Autodesk Fusion 360 part; units mm, degrees
note: some values were not read from the file. Set by a fixed rule: which sketch regions a step uses.
(part 2 of 3)
  line L723 (-61, -7.5056) -> (-66, -4.6188)
  line L724 (-61, -13.2791) -> (-61, -7.5056)
  line L725 (-71, -7.5056) -> (-71, -13.2791)
  line L726 (-71, -13.2791) -> (-66, -16.1658)
  line L727 (-66, -16.1658) -> (-61, -13.2791)
  line L728 (-54, -4.6188) -> (-59, -7.5056)
  line L729 (-49, -7.5056) -> (-54, -4.6188)
  line L730 (-49, -13.2791) -> (-49, -7.5056)
  line L731 (-59, -7.5056) -> (-59, -13.2791)
  line L732 (-59, -13.2791) -> (-54, -16.1658)
  line L733 (-54, -16.1658) -> (-49, -13.2791)
  line L734 (-42, -4.6188) -> (-47, -7.5056)
  line L735 (-37, -7.5056) -> (-42, -4.6188)
  line L736 (-37, -13.2791) -> (-37, -7.5056)
  line L737 (-47, -7.5056) -> (-47, -13.2791)
  line L738 (-47, -13.2791) -> (-42, -16.1658)
  line L739 (-42, -16.1658) -> (-37, -13.2791)
  line L740 (-30, -4.6188) -> (-35, -7.5056)
  line L741 (-25, -7.5056) -> (-30, -4.6188)
  line L742 (-25, -13.2791) -> (-25, -7.5056)
  line L743 (-35, -7.5056) -> (-35, -13.2791)
  line L744 (-35, -13.2791) -> (-30, -16.1658)
  line L745 (-30, -16.1658) -> (-25, -13.2791)
  line L746 (-18, -4.6188) -> (-23, -7.5056)
  line L747 (-13, -7.5056) -> (-18, -4.6188)
  line L748 (-13, -13.2791) -> (-13, -7.5056)
  line L749 (-23, -7.5056) -> (-23, -13.2791)
  line L750 (-23, -13.2791) -> (-18, -16.1658)
  line L751 (-18, -16.1658) -> (-13, -13.2791)
  line L752 (-6, -4.6188) -> (-11, -7.5056)
  line L753 (-1, -7.5056) -> (-6, -4.6188)
  line L754 (-1, -13.2791) -> (-1, -7.5056)
  line L755 (-11, -7.5056) -> (-11, -13.2791)
  line L756 (-11, -13.2791) -> (-6, -16.1658)
  line L757 (-6, -16.1658) -> (-1, -13.2791)
  line L758 (6, -4.6188) -> (1, -7.5056)
  line L759 (11, -7.5056) -> (6, -4.6188)
  line L760 (11, -13.2791) -> (11, -7.5056)
  line L761 (1, -7.5056) -> (1, -13.2791)
  line L762 (1, -13.2791) -> (6, -16.1658)
  line L763 (6, -16.1658) -> (11, -13.2791)
  line L764 (18, -4.6188) -> (13, -7.5056)
  line L765 (23, -7.5056) -> (18, -4.6188)
  line L766 (23, -13.2791) -> (23, -7.5056)
  line L767 (13, -7.5056) -> (13, -13.2791)
  line L768 (13, -13.2791) -> (18, -16.1658)
  line L769 (18, -16.1658) -> (23, -13.2791)
  line L770 (30, -4.6188) -> (25, -7.5056)
  line L771 (35, -7.5056) -> (30, -4.6188)
  line L772 (35, -13.2791) -> (35, -7.5056)
  line L773 (25, -7.5056) -> (25, -13.2791)
  line L774 (25, -13.2791) -> (30, -16.1658)
  line L775 (30, -16.1658) -> (35, -13.2791)
  line L776 (42, -4.6188) -> (37, -7.5056)
  line L777 (47, -7.5056) -> (42, -4.6188)
  line L778 (47, -13.2791) -> (47, -7.5056)
  line L779 (37, -7.5056) -> (37, -13.2791)
  line L780 (37, -13.2791) -> (42, -16.1658)
  line L781 (42, -16.1658) -> (47, -13.2791)
  line L782 (54, -4.6188) -> (49, -7.5056)
  line L783 (59, -7.5056) -> (54, -4.6188)
  line L784 (59, -13.2791) -> (59, -7.5056)
  line L785 (49, -7.5056) -> (49, -13.2791)
  line L786 (49, -13.2791) -> (54, -16.1658)
  line L787 (54, -16.1658) -> (59, -13.2791)
  line L788 (66, -4.6188) -> (61, -7.5056)
  line L789 (71, -7.5056) -> (66, -4.6188)
  line L790 (71, -13.2791) -> (71, -7.5056)
  line L791 (61, -7.5056) -> (61, -13.2791)
  line L792 (61, -13.2791) -> (66, -16.1658)
  line L793 (66, -16.1658) -> (71, -13.2791)
  line L794 (78, -4.6188) -> (73, -7.5056)
  line L795 (83, -7.5056) -> (78, -4.6188)
  line L796 (83, -13.2791) -> (83, -7.5056)
  line L797 (73, -7.5056) -> (73, -13.2791)
  line L798 (73, -13.2791) -> (78, -16.1658)
  line L799 (78, -16.1658) -> (83, -13.2791)
  line L800 (90, -4.6188) -> (85, -7.5056)
  line L801 (95, -7.5056) -> (90, -4.6188)
  line L802 (95, -13.2791) -> (95, -7.5056)
  line L803 (85, -7.5056) -> (85, -13.2791)
  line L804 (85, -13.2791) -> (90, -16.1658)
  line L805 (90, -16.1658) -> (95, -13.2791)
  line L806 (102, -4.6188) -> (97, -7.5056)
  line L807 (107, -7.5056) -> (102, -4.6188)
  line L808 (107, -13.2791) -> (107, -7.5056)
  line L809 (97, -7.5056) -> (97, -13.2791)
  line L810 (97, -13.2791) -> (102, -16.1658)
  line L811 (102, -16.1658) -> (107, -13.2791)
  line L812 (-108, 5.7735) -> (-113, 2.8868)
  line L813 (-103, 2.8868) -> (-108, 5.7735)
  line L814 (-103, -2.8868) -> (-103, 2.8868)
  line L815 (-113, 2.8868) -> (-113, -2.8868)
  line L816 (-113, -2.8868) -> (-108, -5.7735)
  line L817 (-108, -5.7735) -> (-103, -2.8868)
  line L818 (-96, 5.7735) -> (-101, 2.8868)
  line L819 (-91, 2.8868) -> (-96, 5.7735)
  line L820 (-91, -2.8868) -> (-91, 2.8868)
  line L821 (-101, 2.8868) -> (-101, -2.8868)
  line L822 (-101, -2.8868) -> (-96, -5.7735)
  line L823 (-96, -5.7735) -> (-91, -2.8868)
  line L824 (-84, 5.7735) -> (-89, 2.8868)
  line L825 (-79, 2.8868) -> (-84, 5.7735)
  line L826 (-79, -2.8868) -> (-79, 2.8868)
  line L827 (-89, 2.8868) -> (-89, -2.8868)
  line L828 (-89, -2.8868) -> (-84, -5.7735)
  line L829 (-84, -5.7735) -> (-79, -2.8868)
  line L830 (-72, 5.7735) -> (-77, 2.8868)
  line L831 (-67, 2.8868) -> (-72, 5.7735)
  line L832 (-67, -2.8868) -> (-67, 2.8868)
  line L833 (-77, 2.8868) -> (-77, -2.8868)
  line L834 (-77, -2.8868) -> (-72, -5.7735)
  line L835 (-72, -5.7735) -> (-67, -2.8868)
  line L836 (-60, 5.7735) -> (-65, 2.8868)
  line L837 (-55, 2.8868) -> (-60, 5.7735)
  line L838 (-55, -2.8868) -> (-55, 2.8868)
  line L839 (-65, 2.8868) -> (-65, -2.8868)
  line L840 (-65, -2.8868) -> (-60, -5.7735)
  line L841 (-60, -5.7735) -> (-55, -2.8868)
  line L842 (-48, 5.7735) -> (-53, 2.8868)
  line L843 (-43, 2.8868) -> (-48, 5.7735)
  line L844 (-43, -2.8868) -> (-43, 2.8868)
  line L845 (-53, 2.8868) -> (-53, -2.8868)
  line L846 (-53, -2.8868) -> (-48, -5.7735)
  line L847 (-48, -5.7735) -> (-43, -2.8868)
  line L848 (-36, 5.7735) -> (-41, 2.8868)
  line L849 (-31, 2.8868) -> (-36, 5.7735)
  line L850 (-31, -2.8868) -> (-31, 2.8868)
  line L851 (-41, 2.8868) -> (-41, -2.8868)
  line L852 (-41, -2.8868) -> (-36, -5.7735)
  line L853 (-36, -5.7735) -> (-31, -2.8868)
  line L854 (-24, 5.7735) -> (-29, 2.8868)
  line L855 (-19, 2.8868) -> (-24, 5.7735)
  line L856 (-19, -2.8868) -> (-19, 2.8868)
  line L857 (-29, 2.8868) -> (-29, -2.8868)
  line L858 (-29, -2.8868) -> (-24, -5.7735)
  line L859 (-24, -5.7735) -> (-19, -2.8868)
  line L860 (-12, 5.7735) -> (-17, 2.8868)
  line L861 (-7, 2.8868) -> (-12, 5.7735)
  line L862 (-7, -2.8868) -> (-7, 2.8868)
  line L863 (-17, 2.8868) -> (-17, -2.8868)
  line L864 (-17, -2.8868) -> (-12, -5.7735)
  line L865 (-12, -5.7735) -> (-7, -2.8868)
  line L866 (12, 5.7735) -> (7, 2.8868)
  line L867 (17, 2.8868) -> (12, 5.7735)
  line L868 (17, -2.8868) -> (17, 2.8868)
  line L869 (7, 2.8868) -> (7, -2.8868)
  line L870 (7, -2.8868) -> (12, -5.7735)
  line L871 (12, -5.7735) -> (17, -2.8868)
  line L872 (24, 5.7735) -> (19, 2.8868)
  line L873 (29, 2.8868) -> (24, 5.7735)
  line L874 (29, -2.8868) -> (29, 2.8868)
  line L875 (19, 2.8868) -> (19, -2.8868)
  line L876 (19, -2.8868) -> (24, -5.7735)
  line L877 (24, -5.7735) -> (29, -2.8868)
  line L878 (36, 5.7735) -> (31, 2.8868)
  line L879 (41, 2.8868) -> (36, 5.7735)
  line L880 (41, -2.8868) -> (41, 2.8868)
  line L881 (31, 2.8868) -> (31, -2.8868)
  line L882 (31, -2.8868) -> (36, -5.7735)
  line L883 (36, -5.7735) -> (41, -2.8868)
  line L884 (48, 5.7735) -> (43, 2.8868)
  line L885 (53, 2.8868) -> (48, 5.7735)
  line L886 (53, -2.8868) -> (53, 2.8868)
  line L887 (43, 2.8868) -> (43, -2.8868)
  line L888 (43, -2.8868) -> (48, -5.7735)
  line L889 (48, -5.7735) -> (53, -2.8868)
  line L890 (60, 5.7735) -> (55, 2.8868)
  line L891 (65, 2.8868) -> (60, 5.7735)
  line L892 (65, -2.8868) -> (65, 2.8868)
  line L893 (55, 2.8868) -> (55, -2.8868)
  line L894 (55, -2.8868) -> (60, -5.7735)
  line L895 (60, -5.7735) -> (65, -2.8868)
  line L896 (72, 5.7735) -> (67, 2.8868)
  line L897 (77, 2.8868) -> (72, 5.7735)
  line L898 (77, -2.8868) -> (77, 2.8868)
  line L899 (67, 2.8868) -> (67, -2.8868)
  line L900 (67, -2.8868) -> (72, -5.7735)
  line L901 (72, -5.7735) -> (77, -2.8868)
  line L902 (84, 5.7735) -> (79, 2.8868)
  line L903 (89, 2.8868) -> (84, 5.7735)
  line L904 (89, -2.8868) -> (89, 2.8868)
  line L905 (79, 2.8868) -> (79, -2.8868)
  line L906 (79, -2.8868) -> (84, -5.7735)
  line L907 (84, -5.7735) -> (89, -2.8868)
  line L908 (96, 5.7735) -> (91, 2.8868)
  line L909 (101, 2.8868) -> (96, 5.7735)
  line L910 (101, -2.8868) -> (101, 2.8868)
  line L911 (91, 2.8868) -> (91, -2.8868)
  line L912 (91, -2.8868) -> (96, -5.7735)
  line L913 (96, -5.7735) -> (101, -2.8868)
  line L914 (108, 5.7735) -> (103, 2.8868)
  line L915 (113, 2.8868) -> (108, 5.7735)
  line L916 (113, -2.8868) -> (113, 2.8868)
  line L917 (103, 2.8868) -> (103, -2.8868)
  line L918 (103, -2.8868) -> (108, -5.7735)
  line L919 (108, -5.7735) -> (113, -2.8868)
  line L920 (-102, 16.1658) -> (-107, 13.2791)
  line L921 (-97, 13.2791) -> (-102, 16.1658)
  line L922 (-97, 7.5056) -> (-97, 13.2791)
  line L923 (-107, 13.2791) -> (-107, 7.5056)
  line L924 (-107, 7.5056) -> (-102, 4.6188)
  line L925 (-102, 4.6188) -> (-97, 7.5056)
  line L926 (-90, 16.1658) -> (-95, 13.2791)
  line L927 (-85, 13.2791) -> (-90, 16.1658)
  line L928 (-85, 7.5056) -> (-85, 13.2791)
  line L929 (-95, 13.2791) -> (-95, 7.5056)
  line L930 (-95, 7.5056) -> (-90, 4.6188)
  line L931 (-90, 4.6188) -> (-85, 7.5056)
  line L932 (-78, 16.1658) -> (-83, 13.2791)
  line L933 (-73, 13.2791) -> (-78, 16.1658)
  line L934 (-73, 7.5056) -> (-73, 13.2791)
  line L935 (-83, 13.2791) -> (-83, 7.5056)
  line L936 (-83, 7.5056) -> (-78, 4.6188)
  line L937 (-78, 4.6188) -> (-73, 7.5056)
  line L938 (-66, 16.1658) -> (-71, 13.2791)
  line L939 (-61, 13.2791) -> (-66, 16.1658)
  line L940 (-61, 7.5056) -> (-61, 13.2791)
  line L941 (-71, 13.2791) -> (-71, 7.5056)
  line L942 (-71, 7.5056) -> (-66, 4.6188)
  line L943 (-66, 4.6188) -> (-61, 7.5056)
  line L944 (-54, 16.1658) -> (-59, 13.2791)
  line L945 (-49, 13.2791) -> (-54, 16.1658)
  line L946 (-49, 7.5056) -> (-49, 13.2791)
  line L947 (-59, 13.2791) -> (-59, 7.5056)
  line L948 (-59, 7.5056) -> (-54, 4.6188)
  line L949 (-54, 4.6188) -> (-49, 7.5056)
  line L950 (-42, 16.1658) -> (-47, 13.2791)
  line L951 (-37, 13.2791) -> (-42, 16.1658)
  line L952 (-37, 7.5056) -> (-37, 13.2791)
  line L953 (-47, 13.2791) -> (-47, 7.5056)
  line L954 (-47, 7.5056) -> (-42, 4.6188)
  line L955 (-42, 4.6188) -> (-37, 7.5056)
  line L956 (-30, 16.1658) -> (-35, 13.2791)
  line L957 (-25, 13.2791) -> (-30, 16.1658)
  line L958 (-25, 7.5056) -> (-25, 13.2791)
  line L959 (-35, 13.2791) -> (-35, 7.5056)
  line L960 (-35, 7.5056) -> (-30, 4.6188)
  line L961 (-30, 4.6188) -> (-25, 7.5056)
  line L962 (-18, 16.1658) -> (-23, 13.2791)
  line L963 (-13, 13.2791) -> (-18, 16.1658)
  line L964 (-13, 7.5056) -> (-13, 13.2791)
  line L965 (-23, 13.2791) -> (-23, 7.5056)
  line L966 (-23, 7.5056) -> (-18, 4.6188)
  line L967 (-18, 4.6188) -> (-13, 7.5056)
  line L968 (-6, 16.1658) -> (-11, 13.2791)
  line L969 (-1, 13.2791) -> (-6, 16.1658)
  line L970 (-1, 7.5056) -> (-1, 13.2791)
  line L971 (-11, 13.2791) -> (-11, 7.5056)
  line L972 (-11, 7.5056) -> (-6, 4.6188)
  line L973 (-6, 4.6188) -> (-1, 7.5056)
  line L974 (6, 16.1658) -> (1, 13.2791)
  line L975 (11, 13.2791) -> (6, 16.1658)
  line L976 (11, 7.5056) -> (11, 13.2791)
  line L977 (1, 13.2791) -> (1, 7.5056)
  line L978 (1, 7.5056) -> (6, 4.6188)
  line L979 (6, 4.6188) -> (11, 7.5056)
  line L980 (18, 16.1658) -> (13, 13.2791)
  line L981 (23, 13.2791) -> (18, 16.1658)
  line L982 (23, 7.5056) -> (23, 13.2791)
  line L983 (13, 13.2791) -> (13, 7.5056)
  line L984 (13, 7.5056) -> (18, 4.6188)
  line L985 (18, 4.6188) -> (23, 7.5056)
  line L986 (30, 16.1658) -> (25, 13.2791)
  line L987 (35, 13.2791) -> (30, 16.1658)
  line L988 (35, 7.5056) -> (35, 13.2791)
  line L989 (25, 13.2791) -> (25, 7.5056)
  line L990 (25, 7.5056) -> (30, 4.6188)
  line L991 (30, 4.6188) -> (35, 7.5056)
  line L992 (42, 16.1658) -> (37, 13.2791)
  line L993 (47, 13.2791) -> (42, 16.1658)
  line L994 (47, 7.5056) -> (47, 13.2791)
  line L995 (37, 13.2791) -> (37, 7.5056)
  line L996 (37, 7.5056) -> (42, 4.6188)
  line L997 (42, 4.6188) -> (47, 7.5056)
  line L998 (54, 16.1658) -> (49, 13.2791)
  line L999 (59, 13.2791) -> (54, 16.1658)
  line L1000 (59, 7.5056) -> (59, 13.2791)
  line L1001 (49, 13.2791) -> (49, 7.5056)
  line L1002 (49, 7.5056) -> (54, 4.6188)
  line L1003 (54, 4.6188) -> (59, 7.5056)
  line L1004 (66, 16.1658) -> (61, 13.2791)
  line L1005 (71, 13.2791) -> (66, 16.1658)
  line L1006 (71, 7.5056) -> (71, 13.2791)
  line L1007 (61, 13.2791) -> (61, 7.5056)
  line L1008 (61, 7.5056) -> (66, 4.6188)
  line L1009 (66, 4.6188) -> (71, 7.5056)
  line L1010 (78, 16.1658) -> (73, 13.2791)
  line L1011 (83, 13.2791) -> (78, 16.1658)
  line L1012 (83, 7.5056) -> (83, 13.2791)
  line L1013 (73, 13.2791) -> (73, 7.5056)
  line L1014 (73, 7.5056) -> (78, 4.6188)
  line L1015 (78, 4.6188) -> (83, 7.5056)
  line L1016 (90, 16.1658) -> (85, 13.2791)
  line L1017 (95, 13.2791) -> (90, 16.1658)
  line L1018 (95, 7.5056) -> (95, 13.2791)
  line L1019 (85, 13.2791) -> (85, 7.5056)
  line L1020 (85, 7.5056) -> (90, 4.6188)
  line L1021 (90, 4.6188) -> (95, 7.5056)
  line L1022 (102, 16.1658) -> (97, 13.2791)
  line L1023 (107, 13.2791) -> (102, 16.1658)
  line L1024 (107, 7.5056) -> (107, 13.2791)
  line L1025 (97, 13.2791) -> (97, 7.5056)
  line L1026 (97, 7.5056) -> (102, 4.6188)
  line L1027 (102, 4.6188) -> (107, 7.5056)
  line L1028 (114, 16.1658) -> (109, 13.2791)
  line L1029 (119, 13.2791) -> (114, 16.1658)
  line L1030 (119, 7.5056) -> (119, 13.2791)
  line L1031 (109, 13.2791) -> (109, 7.5056)
  line L1032 (109, 7.5056) -> (114, 4.6188)
  line L1033 (114, 4.6188) -> (119, 7.5056)
  line L1034 (-96, 26.5581) -> (-101, 23.6714)
  line L1035 (-91, 23.6714) -> (-96, 26.5581)
  line L1036 (-91, 17.8979) -> (-91, 23.6714)
  line L1037 (-101, 23.6714) -> (-101, 17.8979)
  line L1038 (-101, 17.8979) -> (-96, 15.0111)
  line L1039 (-96, 15.0111) -> (-91, 17.8979)
  line L1040 (-84, 26.5581) -> (-89, 23.6714)
  line L1041 (-79, 23.6714) -> (-84, 26.5581)
  line L1042 (-79, 17.8979) -> (-79, 23.6714)
  line L1043 (-89, 23.6714) -> (-89, 17.8979)
  line L1044 (-89, 17.8979) -> (-84, 15.0111)
  line L1045 (-84, 15.0111) -> (-79, 17.8979)
  line L1046 (-72, 26.5581) -> (-77, 23.6714)
  line L1047 (-67, 23.6714) -> (-72, 26.5581)
  line L1048 (-67, 17.8979) -> (-67, 23.6714)
  line L1049 (-77, 23.6714) -> (-77, 17.8979)
  line L1050 (-77, 17.8979) -> (-72, 15.0111)
  line L1051 (-72, 15.0111) -> (-67, 17.8979)
  line L1052 (-60, 26.5581) -> (-65, 23.6714)
  line L1053 (-55, 23.6714) -> (-60, 26.5581)
  line L1054 (-55, 17.8979) -> (-55, 23.6714)
  line L1055 (-65, 23.6714) -> (-65, 17.8979)
  line L1056 (-65, 17.8979) -> (-60, 15.0111)
  line L1057 (-60, 15.0111) -> (-55, 17.8979)
  line L1058 (-48, 26.5581) -> (-53, 23.6714)
  line L1059 (-43, 23.6714) -> (-48, 26.5581)
  line L1060 (-43, 17.8979) -> (-43, 23.6714)
  line L1061 (-53, 23.6714) -> (-53, 17.8979)
  line L1062 (-53, 17.8979) -> (-48, 15.0111)
  line L1063 (-48, 15.0111) -> (-43, 17.8979)
  line L1064 (-36, 26.5581) -> (-41, 23.6714)
  line L1065 (-31, 23.6714) -> (-36, 26.5581)
  line L1066 (-31, 17.8979) -> (-31, 23.6714)
  line L1067 (-41, 23.6714) -> (-41, 17.8979)
  line L1068 (-41, 17.8979) -> (-36, 15.0111)
  line L1069 (-36, 15.0111) -> (-31, 17.8979)
  line L1070 (-24, 26.5581) -> (-29, 23.6714)
  line L1071 (-19, 23.6714) -> (-24, 26.5581)
  line L1072 (-19, 17.8979) -> (-19, 23.6714)
  line L1073 (-29, 23.6714) -> (-29, 17.8979)
  line L1074 (-29, 17.8979) -> (-24, 15.0111)
  line L1075 (-24, 15.0111) -> (-19, 17.8979)
  line L1076 (-12, 26.5581) -> (-17, 23.6714)
  line L1077 (-7, 23.6714) -> (-12, 26.5581)
  line L1078 (-7, 17.8979) -> (-7, 23.6714)
  line L1079 (-17, 23.6714) -> (-17, 17.8979)
  line L1080 (-17, 17.8979) -> (-12, 15.0111)
  line L1081 (-12, 15.0111) -> (-7, 17.8979)
  line L1082 (0, 26.5581) -> (-5, 23.6714)
  line L1083 (5, 23.6714) -> (0, 26.5581)
  line L1084 (5, 17.8979) -> (5, 23.6714)
  line L1085 (-5, 23.6714) -> (-5, 17.8979)
  line L1086 (-5, 17.8979) -> (0, 15.0111)
  line L1087 (0, 15.0111) -> (5, 17.8979)
  line L1088 (12, 26.5581) -> (7, 23.6714)
  line L1089 (17, 23.6714) -> (12, 26.5581)
  line L1090 (17, 17.8979) -> (17, 23.6714)
  line L1091 (7, 23.6714) -> (7, 17.8979)
  line L1092 (7, 17.8979) -> (12, 15.0111)
  line L1093 (12, 15.0111) -> (17, 17.8979)
  line L1094 (24, 26.5581) -> (19, 23.6714)
  line L1095 (29, 23.6714) -> (24, 26.5581)
  line L1096 (29, 17.8979) -> (29, 23.6714)
  line L1097 (19, 23.6714) -> (19, 17.8979)
  line L1098 (19, 17.8979) -> (24, 15.0111)
  line L1099 (24, 15.0111) -> (29, 17.8979)
  line L1100 (36, 26.5581) -> (31, 23.6714)
  line L1101 (41, 23.6714) -> (36, 26.5581)
  line L1102 (41, 17.8979) -> (41, 23.6714)
  line L1103 (31, 23.6714) -> (31, 17.8979)
  line L1104 (31, 17.8979) -> (36, 15.0111)
  line L1105 (36, 15.0111) -> (41, 17.8979)
  line L1106 (48, 26.5581) -> (43, 23.6714)
  line L1107 (53, 23.6714) -> (48, 26.5581)
  line L1108 (53, 17.8979) -> (53, 23.6714)
  line L1109 (43, 23.6714) -> (43, 17.8979)
  line L1110 (43, 17.8979) -> (48, 15.0111)
  line L1111 (48, 15.0111) -> (53, 17.8979)
  line L1112 (60, 26.5581) -> (55, 23.6714)
  line L1113 (65, 23.6714) -> (60, 26.5581)
  line L1114 (65, 17.8979) -> (65, 23.6714)
  line L1115 (55, 23.6714) -> (55, 17.8979)
  line L1116 (55, 17.8979) -> (60, 15.0111)
  line L1117 (60, 15.0111) -> (65, 17.8979)
  line L1118 (72, 26.5581) -> (67, 23.6714)
  line L1119 (77, 23.6714) -> (72, 26.5581)
  line L1120 (77, 17.8979) -> (77, 23.6714)
  line L1121 (67, 23.6714) -> (67, 17.8979)
  line L1122 (67, 17.8979) -> (72, 15.0111)
  line L1123 (72, 15.0111) -> (77, 17.8979)
  line L1124 (84, 26.5581) -> (79, 23.6714)
  line L1125 (89, 23.6714) -> (84, 26.5581)
  line L1126 (89, 17.8979) -> (89, 23.6714)
  line L1127 (79, 23.6714) -> (79, 17.8979)
  line L1128 (79, 17.8979) -> (84, 15.0111)
  line L1129 (84, 15.0111) -> (89, 17.8979)
  line L1130 (96, 26.5581) -> (91, 23.6714)
  line L1131 (101, 23.6714) -> (96, 26.5581)
  line L1132 (101, 17.8979) -> (101, 23.6714)
  line L1133 (91, 23.6714) -> (91, 17.8979)
  line L1134 (91, 17.8979) -> (96, 15.0111)
  line L1135 (96, 15.0111) -> (101, 17.8979)
  line L1136 (108, 26.5581) -> (103, 23.6714)
  line L1137 (113, 23.6714) -> (108, 26.5581)
  line L1138 (113, 17.8979) -> (113, 23.6714)
  line L1139 (103, 23.6714) -> (103, 17.8979)
  line L1140 (103, 17.8979) -> (108, 15.0111)
  line L1141 (108, 15.0111) -> (113, 17.8979)
  line L1142 (120, 26.5581) -> (115, 23.6714)
  line L1143 (125, 23.6714) -> (120, 26.5581)
  line L1144 (125, 17.8979) -> (125, 23.6714)
  line L1145 (115, 23.6714) -> (115, 17.8979)
  line L1146 (115, 17.8979) -> (120, 15.0111)
  line L1147 (120, 15.0111) -> (125, 17.8979)
  line L1148 (-90, 36.9504) -> (-95, 34.0637)
  line L1149 (-85, 34.0637) -> (-90, 36.9504)
  line L1150 (-85, 28.2902) -> (-85, 34.0637)
  line L1151 (-95, 34.0637) -> (-95, 28.2902)
  line L1152 (-95, 28.2902) -> (-90, 25.4034)
  line L1153 (-90, 25.4034) -> (-85, 28.2902)
  line L1154 (-78, 36.9504) -> (-83, 34.0637)
  line L1155 (-73, 34.0637) -> (-78, 36.9504)
  line L1156 (-73, 28.2902) -> (-73, 34.0637)
  line L1157 (-83, 34.0637) -> (-83, 28.2902)
  line L1158 (-83, 28.2902) -> (-78, 25.4034)
  line L1159 (-78, 25.4034) -> (-73, 28.2902)
  line L1160 (-66, 36.9504) -> (-71, 34.0637)
  line L1161 (-61, 34.0637) -> (-66, 36.9504)
  line L1162 (-61, 28.2902) -> (-61, 34.0637)
  line L1163 (-71, 34.0637) -> (-71, 28.2902)
  line L1164 (-71, 28.2902) -> (-66, 25.4034)
  line L1165 (-66, 25.4034) -> (-61, 28.2902)
  line L1166 (-54, 36.9504) -> (-59, 34.0637)
  line L1167 (-49, 34.0637) -> (-54, 36.9504)
  line L1168 (-49, 28.2902) -> (-49, 34.0637)
  line L1169 (-59, 34.0637) -> (-59, 28.2902)
  line L1170 (-59, 28.2902) -> (-54, 25.4034)
  line L1171 (-54, 25.4034) -> (-49, 28.2902)
  line L1172 (-42, 36.9504) -> (-47, 34.0637)
  line L1173 (-37, 34.0637) -> (-42, 36.9504)
  line L1174 (-37, 28.2902) -> (-37, 34.0637)
  line L1175 (-47, 34.0637) -> (-47, 28.2902)
  line L1176 (-47, 28.2902) -> (-42, 25.4034)
  line L1177 (-42, 25.4034) -> (-37, 28.2902)
  line L1178 (-30, 36.9504) -> (-35, 34.0637)
  line L1179 (-25, 34.0637) -> (-30, 36.9504)
  line L1180 (-25, 28.2902) -> (-25, 34.0637)
  line L1181 (-35, 34.0637) -> (-35, 28.2902)
  line L1182 (-35, 28.2902) -> (-30, 25.4034)
  line L1183 (-30, 25.4034) -> (-25, 28.2902)
  line L1184 (-18, 36.9504) -> (-23, 34.0637)
  line L1185 (-13, 34.0637) -> (-18, 36.9504)
  line L1186 (-13, 28.2902) -> (-13, 34.0637)
  line L1187 (-23, 34.0637) -> (-23, 28.2902)
  line L1188 (-23, 28.2902) -> (-18, 25.4034)
  line L1189 (-18, 25.4034) -> (-13, 28.2902)
  line L1190 (-6, 36.9504) -> (-11, 34.0637)
  line L1191 (-1, 34.0637) -> (-6, 36.9504)
  line L1192 (-1, 28.2902) -> (-1, 34.0637)
  line L1193 (-11, 34.0637) -> (-11, 28.2902)
  line L1194 (-11, 28.2902) -> (-6, 25.4034)
  line L1195 (-6, 25.4034) -> (-1, 28.2902)
  line L1196 (6, 36.9504) -> (1, 34.0637)
  line L1197 (11, 34.0637) -> (6, 36.9504)
  line L1198 (11, 28.2902) -> (11, 34.0637)
  line L1199 (1, 34.0637) -> (1, 28.2902)
  line L1200 (1, 28.2902) -> (6, 25.4034)
  line L1201 (6, 25.4034) -> (11, 28.2902)
  line L1202 (18, 36.9504) -> (13, 34.0637)
  line L1203 (23, 34.0637) -> (18, 36.9504)
  line L1204 (23, 28.2902) -> (23, 34.0637)
  line L1205 (13, 34.0637) -> (13, 28.2902)
  line L1206 (13, 28.2902) -> (18, 25.4034)
  line L1207 (18, 25.4034) -> (23, 28.2902)
  line L1208 (30, 36.9504) -> (25, 34.0637)
  line L1209 (35, 34.0637) -> (30, 36.9504)
  line L1210 (35, 28.2902) -> (35, 34.0637)
  line L1211 (25, 34.0637) -> (25, 28.2902)
  line L1212 (25, 28.2902) -> (30, 25.4034)
  line L1213 (30, 25.4034) -> (35, 28.2902)
  line L1214 (42, 36.9504) -> (37, 34.0637)
  line L1215 (47, 34.0637) -> (42, 36.9504)
  line L1216 (47, 28.2902) -> (47, 34.0637)
  line L1217 (37, 34.0637) -> (37, 28.2902)
  line L1218 (37, 28.2902) -> (42, 25.4034)
  line L1219 (42, 25.4034) -> (47, 28.2902)
  line L1220 (54, 36.9504) -> (49, 34.0637)
  line L1221 (59, 34.0637) -> (54, 36.9504)
  line L1222 (59, 28.2902) -> (59, 34.0637)
  line L1223 (49, 34.0637) -> (49, 28.2902)
  line L1224 (49, 28.2902) -> (54, 25.4034)
  line L1225 (54, 25.4034) -> (59, 28.2902)
  line L1226 (66, 36.9504) -> (61, 34.0637)
  line L1227 (71, 34.0637) -> (66, 36.9504)
  line L1228 (71, 28.2902) -> (71, 34.0637)
  line L1229 (61, 34.0637) -> (61, 28.2902)
  line L1230 (61, 28.2902) -> (66, 25.4034)
  line L1231 (66, 25.4034) -> (71, 28.2902)
  line L1232 (78, 36.9504) -> (73, 34.0637)
  line L1233 (83, 34.0637) -> (78, 36.9504)
  line L1234 (83, 28.2902) -> (83, 34.0637)
  line L1235 (73, 34.0637) -> (73, 28.2902)
  line L1236 (73, 28.2902) -> (78, 25.4034)
  line L1237 (78, 25.4034) -> (83, 28.2902)
  line L1238 (90, 36.9504) -> (85, 34.0637)
  line L1239 (95, 34.0637) -> (90, 36.9504)
  line L1240 (95, 28.2902) -> (95, 34.0637)
  line L1241 (85, 34.0637) -> (85, 28.2902)
  line L1242 (85, 28.2902) -> (90, 25.4034)
  line L1243 (90, 25.4034) -> (95, 28.2902)
  line L1244 (102, 36.9504) -> (97, 34.0637)
  line L1245 (107, 34.0637) -> (102, 36.9504)
  line L1246 (107, 28.2902) -> (107, 34.0637)
  line L1247 (97, 34.0637) -> (97, 28.2902)
  line L1248 (97, 28.2902) -> (102, 25.4034)
  line L1249 (102, 25.4034) -> (107, 28.2902)
  line L1250 (114, 36.9504) -> (109, 34.0637)
  line L1251 (119, 34.0637) -> (114, 36.9504)
  line L1252 (119, 28.2902) -> (119, 34.0637)
  line L1253 (109, 34.0637) -> (109, 28.2902)
  line L1254 (109, 28.2902) -> (114, 25.4034)
  line L1255 (114, 25.4034) -> (119, 28.2902)
  line L1256 (126, 36.9504) -> (121, 34.0637)
  line L1257 (131, 34.0637) -> (126, 36.9504)
  line L1258 (131, 28.2902) -> (131, 34.0637)
  line L1259 (121, 34.0637) -> (121, 28.2902)
  line L1260 (121, 28.2902) -> (126, 25.4034)
  line L1261 (126, 25.4034) -> (131, 28.2902)
  line L1262 (-84, 47.3427) -> (-89, 44.456)
  line L1263 (-79, 44.456) -> (-84, 47.3427)
  line L1264 (-79, 38.6825) -> (-79, 44.456)
  line L1265 (-89, 44.456) -> (-89, 38.6825)
  line L1266 (-89, 38.6825) -> (-84, 35.7957)
  line L1267 (-84, 35.7957) -> (-79, 38.6825)
  line L1268 (-72, 47.3427) -> (-77, 44.456)
  line L1269 (-67, 44.456) -> (-72, 47.3427)
  line L1270 (-67, 38.6825) -> (-67, 44.456)
  line L1271 (-77, 44.456) -> (-77, 38.6825)
  line L1272 (-77, 38.6825) -> (-72, 35.7957)
  line L1273 (-72, 35.7957) -> (-67, 38.6825)
  line L1274 (-60, 47.3427) -> (-65, 44.456)
  line L1275 (-55, 44.456) -> (-60, 47.3427)
  line L1276 (-55, 38.6825) -> (-55, 44.456)
  line L1277 (-65, 44.456) -> (-65, 38.6825)
  line L1278 (-65, 38.6825) -> (-60, 35.7957)
  line L1279 (-60, 35.7957) -> (-55, 38.6825)
  line L1280 (-48, 47.3427) -> (-53, 44.456)
  line L1281 (-43, 44.456) -> (-48, 47.3427)
  line L1282 (-43, 38.6825) -> (-43, 44.456)
  line L1283 (-53, 44.456) -> (-53, 38.6825)
  line L1284 (-53, 38.6825) -> (-48, 35.7957)
  line L1285 (-48, 35.7957) -> (-43, 38.6825)
  line L1286 (-36, 47.3427) -> (-41, 44.456)
  line L1287 (-31, 44.456) -> (-36, 47.3427)
  line L1288 (-31, 38.6825) -> (-31, 44.456)
  line L1289 (-41, 44.456) -> (-41, 38.6825)
  line L1290 (-41, 38.6825) -> (-36, 35.7957)
  line L1291 (-36, 35.7957) -> (-31, 38.6825)
  line L1292 (-24, 47.3427) -> (-29, 44.456)
  line L1293 (-19, 44.456) -> (-24, 47.3427)
  line L1294 (-19, 38.6825) -> (-19, 44.456)
  line L1295 (-29, 44.456) -> (-29, 38.6825)
  line L1296 (-29, 38.6825) -> (-24, 35.7957)
  line L1297 (-24, 35.7957) -> (-19, 38.6825)
  line L1298 (-12, 47.3427) -> (-17, 44.456)
  line L1299 (-7, 44.456) -> (-12, 47.3427)
  line L1300 (-7, 38.6825) -> (-7, 44.456)
  line L1301 (-17, 44.456) -> (-17, 38.6825)
  line L1302 (-17, 38.6825) -> (-12, 35.7957)
  line L1303 (-12, 35.7957) -> (-7, 38.6825)
  line L1304 (0, 47.3427) -> (-5, 44.456)
  line L1305 (5, 44.456) -> (0, 47.3427)
  line L1306 (5, 38.6825) -> (5, 44.456)
  line L1307 (-5, 44.456) -> (-5, 38.6825)
  line L1308 (-5, 38.6825) -> (0, 35.7957)
  line L1309 (0, 35.7957) -> (5, 38.6825)
  line L1310 (12, 47.3427) -> (7, 44.456)
  line L1311 (17, 44.456) -> (12, 47.3427)
  line L1312 (17, 38.6825) -> (17, 44.456)
  line L1313 (7, 44.456) -> (7, 38.6825)
  line L1314 (7, 38.6825) -> (12, 35.7957)
  line L1315 (12, 35.7957) -> (17, 38.6825)
  line L1316 (24, 47.3427) -> (19, 44.456)
  line L1317 (29, 44.456) -> (24, 47.3427)
  line L1318 (29, 38.6825) -> (29, 44.456)
  line L1319 (19, 44.456) -> (19, 38.6825)
  line L1320 (19, 38.6825) -> (24, 35.7957)
  line L1321 (24, 35.7957) -> (29, 38.6825)
  line L1322 (36, 47.3427) -> (31, 44.456)
  line L1323 (41, 44.456) -> (36, 47.3427)
  line L1324 (41, 38.6825) -> (41, 44.456)
  line L1325 (31, 44.456) -> (31, 38.6825)
  line L1326 (31, 38.6825) -> (36, 35.7957)
  line L1327 (36, 35.7957) -> (41, 38.6825)
  line L1328 (48, 47.3427) -> (43, 44.456)
  line L1329 (53, 44.456) -> (48, 47.3427)
  line L1330 (53, 38.6825) -> (53, 44.456)
  line L1331 (43, 44.456) -> (43, 38.6825)
  line L1332 (43, 38.6825) -> (48, 35.7957)
  line L1333 (48, 35.7957) -> (53, 38.6825)
  line L1334 (60, 47.3427) -> (55, 44.456)
  line L1335 (65, 44.456) -> (60, 47.3427)
  line L1336 (65, 38.6825) -> (65, 44.456)
  line L1337 (55, 44.456) -> (55, 38.6825)
  line L1338 (55, 38.6825) -> (60, 35.7957)
  line L1339 (60, 35.7957) -> (65, 38.6825)
  line L1340 (72, 47.3427) -> (67, 44.456)
  line L1341 (77, 44.456) -> (72, 47.3427)
  line L1342 (77, 38.6825) -> (77, 44.456)
  line L1343 (67, 44.456) -> (67, 38.6825)
  line L1344 (67, 38.6825) -> (72, 35.7957)
  line L1345 (72, 35.7957) -> (77, 38.6825)
  line L1346 (84, 47.3427) -> (79, 44.456)
  line L1347 (89, 44.456) -> (84, 47.3427)
  line L1348 (89, 38.6825) -> (89, 44.456)
  line L1349 (79, 44.456) -> (79, 38.6825)
  line L1350 (79, 38.6825) -> (84, 35.7957)
  line L1351 (84, 35.7957) -> (89, 38.6825)
  line L1352 (96, 47.3427) -> (91, 44.456)
  line L1353 (101, 44.456) -> (96, 47.3427)
  line L1354 (101, 38.6825) -> (101, 44.456)
  line L1355 (91, 44.456) -> (91, 38.6825)
  line L1356 (91, 38.6825) -> (96, 35.7957)
  line L1357 (96, 35.7957) -> (101, 38.6825)
  line L1358 (108, 47.3427) -> (103, 44.456)
  line L1359 (113, 44.456) -> (108, 47.3427)
  line L1360 (113, 38.6825) -> (113, 44.456)
  line L1361 (103, 44.456) -> (103, 38.6825)
  line L1362 (103, 38.6825) -> (108, 35.7957)
  line L1363 (108, 35.7957) -> (113, 38.6825)
  line L1364 (120, 47.3427) -> (115, 44.456)
  line L1365 (125, 44.456) -> (120, 47.3427)
  line L1366 (125, 38.6825) -> (125, 44.456)
  line L1367 (115, 44.456) -> (115, 38.6825)
  line L1368 (115, 38.6825) -> (120, 35.7957)
  line L1369 (120, 35.7957) -> (125, 38.6825)
  line L1370 (132, 47.3427) -> (127, 44.456)
  line L1371 (137, 44.456) -> (132, 47.3427)
  line L1372 (137, 38.6825) -> (137, 44.456)
  line L1373 (127, 44.456) -> (127, 38.6825)
  line L1374 (127, 38.6825) -> (132, 35.7957)
  line L1375 (132, 35.7957) -> (137, 38.6825)
  line L1376 (-78, 57.735) -> (-83, 54.8483)
  line L1377 (-73, 54.8483) -> (-78, 57.735)
  line L1378 (-73, 49.0748) -> (-73, 54.8483)
  line L1379 (-83, 54.8483) -> (-83, 49.0748)
  line L1380 (-83, 49.0748) -> (-78, 46.188)
  line L1381 (-78, 46.188) -> (-73, 49.0748)
  line L1382 (-66, 57.735) -> (-71, 54.8483)
  line L1383 (-61, 54.8483) -> (-66, 57.735)
  line L1384 (-61, 49.0748) -> (-61, 54.8483)
  line L1385 (-71, 54.8483) -> (-71, 49.0748)
  line L1386 (-71, 49.0748) -> (-66, 46.188)
  line L1387 (-66, 46.188) -> (-61, 49.0748)
  line L1388 (-54, 57.735) -> (-59, 54.8483)
  line L1389 (-49, 54.8483) -> (-54, 57.735)
  line L1390 (-49, 49.0748) -> (-49, 54.8483)
  line L1391 (-59, 54.8483) -> (-59, 49.0748)
  line L1392 (-59, 49.0748) -> (-54, 46.188)
  line L1393 (-54, 46.188) -> (-49, 49.0748)
  line L1394 (-42, 57.735) -> (-47, 54.8483)
  line L1395 (-37, 54.8483) -> (-42, 57.735)
  line L1396 (-37, 49.0748) -> (-37, 54.8483)
  line L1397 (-47, 54.8483) -> (-47, 49.0748)
  line L1398 (-47, 49.0748) -> (-42, 46.188)
  line L1399 (-42, 46.188) -> (-37, 49.0748)
  line L1400 (-30, 57.735) -> (-35, 54.8483)
  line L1401 (-25, 54.8483) -> (-30, 57.735)
  line L1402 (-25, 49.0748) -> (-25, 54.8483)
  line L1403 (-35, 54.8483) -> (-35, 49.0748)
  line L1404 (-35, 49.0748) -> (-30, 46.188)
  line L1405 (-30, 46.188) -> (-25, 49.0748)
  line L1406 (-18, 57.735) -> (-23, 54.8483)
  line L1407 (-13, 54.8483) -> (-18, 57.735)
  line L1408 (-13, 49.0748) -> (-13, 54.8483)
  line L1409 (-23, 54.8483) -> (-23, 49.0748)
  line L1410 (-23, 49.0748) -> (-18, 46.188)
  line L1411 (-18, 46.188) -> (-13, 49.0748)
  line L1412 (-6, 57.735) -> (-11, 54.8483)
  line L1413 (-1, 54.8483) -> (-6, 57.735)
  line L1414 (-1, 49.0748) -> (-1, 54.8483)
  line L1415 (-11, 54.8483) -> (-11, 49.0748)
  line L1416 (-11, 49.0748) -> (-6, 46.188)
  line L1417 (-6, 46.188) -> (-1, 49.0748)
  line L1418 (6, 57.735) -> (1, 54.8483)
  line L1419 (11, 54.8483) -> (6, 57.735)
  line L1420 (11, 49.0748) -> (11, 54.8483)
  line L1421 (1, 54.8483) -> (1, 49.0748)
  line L1422 (1, 49.0748) -> (6, 46.188)
  line L1423 (6, 46.188) -> (11, 49.0748)
  line L1424 (18, 57.735) -> (13, 54.8483)
  line L1425 (23, 54.8483) -> (18, 57.735)
  line L1426 (23, 49.0748) -> (23, 54.8483)
  line L1427 (13, 54.8483) -> (13, 49.0748)
  line L1428 (13, 49.0748) -> (18, 46.188)
  line L1429 (18, 46.188) -> (23, 49.0748)
  line L1430 (30, 57.735) -> (25, 54.8483)
  line L1431 (35, 54.8483) -> (30, 57.735)
  line L1432 (35, 49.0748) -> (35, 54.8483)
  line L1433 (25, 54.8483) -> (25, 49.0748)
  line L1434 (25, 49.0748) -> (30, 46.188)
  line L1435 (30, 46.188) -> (35, 49.0748)
  line L1436 (42, 57.735) -> (37, 54.8483)
  line L1437 (47, 54.8483) -> (42, 57.735)
  line L1438 (47, 49.0748) -> (47, 54.8483)
  line L1439 (37, 54.8483) -> (37, 49.0748)
  line L1440 (37, 49.0748) -> (42, 46.188)
  line L1441 (42, 46.188) -> (47, 49.0748)
  line L1442 (54, 57.735) -> (49, 54.8483)
  line L1443 (59, 54.8483) -> (54, 57.735)
  line L1444 (59, 49.0748) -> (59, 54.8483)
  line L1445 (49, 54.8483) -> (49, 49.0748)
  line L1446 (49, 49.0748) -> (54, 46.188)
  line L1447 (54, 46.188) -> (59, 49.0748)
  line L1448 (66, 57.735) -> (61, 54.8483)
  line L1449 (71, 54.8483) -> (66, 57.735)
  line L1450 (71, 49.0748) -> (71, 54.8483)
  line L1451 (61, 54.8483) -> (61, 49.0748)
  line L1452 (61, 49.0748) -> (66, 46.188)
  line L1453 (66, 46.188) -> (71, 49.0748)
  line L1454 (78, 57.735) -> (73, 54.8483)
  line L1455 (83, 54.8483) -> (78, 57.735)
  line L1456 (83, 49.0748) -> (83, 54.8483)
  line L1457 (73, 54.8483) -> (73, 49.0748)
  line L1458 (73, 49.0748) -> (78, 46.188)
  line L1459 (78, 46.188) -> (83, 49.0748)
  line L1460 (90, 57.735) -> (85, 54.8483)
  line L1461 (95, 54.8483) -> (90, 57.735)
  line L1462 (95, 49.0748) -> (95, 54.8483)
  line L1463 (85, 54.8483) -> (85, 49.0748)
  line L1464 (85, 49.0748) -> (90, 46.188)
  line L1465 (90, 46.188) -> (95, 49.0748)
  line L1466 (102, 57.735) -> (97, 54.8483)
  line L1467 (107, 54.8483) -> (102, 57.735)
  line L1468 (107, 49.0748) -> (107, 54.8483)
  line L1469 (97, 54.8483) -> (97, 49.0748)
  line L1470 (97, 49.0748) -> (102, 46.188)
  line L1471 (102, 46.188) -> (107, 49.0748)
  line L1472 (114, 57.735) -> (109, 54.8483)
  line L1473 (119, 54.8483) -> (114, 57.735)
  line L1474 (119, 49.0748) -> (119, 54.8483)
  line L1475 (109, 54.8483) -> (109, 49.0748)
  line L1476 (109, 49.0748) -> (114, 46.188)
  line L1477 (114, 46.188) -> (119, 49.0748)
  line L1478 (126, 57.735) -> (121, 54.8483)
  line L1479 (131, 54.8483) -> (126, 57.735)
  line L1480 (131, 49.0748) -> (131, 54.8483)
  line L1481 (121, 54.8483) -> (121, 49.0748)
  line L1482 (121, 49.0748) -> (126, 46.188)
  line L1483 (126, 46.188) -> (131, 49.0748)
  line L1484 (138, 57.735) -> (133, 54.8483)
  line L1485 (143, 54.8483) -> (138, 57.735)
  line L1486 (143, 49.0748) -> (143, 54.8483)
  line L1487 (133, 54.8483) -> (133, 49.0748)
  line L1488 (133, 49.0748) -> (138, 46.188)
  line L1489 (138, 46.188) -> (143, 49.0748)
  line L1490 (-72, 68.1273) -> (-77, 65.2406)
  line L1491 (-67, 65.2406) -> (-72, 68.1273)
  line L1492 (-67, 59.4671) -> (-67, 65.2406)
  line L1493 (-77, 65.2406) -> (-77, 59.4671)
  line L1494 (-77, 59.4671) -> (-72, 56.5803)
  line L1495 (-72, 56.5803) -> (-67, 59.4671)
  line L1496 (-60, 68.1273) -> (-65, 65.2406)
  line L1497 (-55, 65.2406) -> (-60, 68.1273)
  line L1498 (-55, 59.4671) -> (-55, 65.2406)
  line L1499 (-65, 65.2406) -> (-65, 59.4671)
  line L1500 (-65, 59.4671) -> (-60, 56.5803)
  line L1501 (-60, 56.5803) -> (-55, 59.4671)
  line L1502 (-48, 68.1273) -> (-53, 65.2406)
  line L1503 (-43, 65.2406) -> (-48, 68.1273)
  line L1504 (-43, 59.4671) -> (-43, 65.2406)
  line L1505 (-53, 65.2406) -> (-53, 59.4671)
  line L1506 (-53, 59.4671) -> (-48, 56.5803)
  line L1507 (-48, 56.5803) -> (-43, 59.4671)
  line L1508 (-36, 68.1273) -> (-41, 65.2406)
  line L1509 (-31, 65.2406) -> (-36, 68.1273)
  line L1510 (-31, 59.4671) -> (-31, 65.2406)
  line L1511 (-41, 65.2406) -> (-41, 59.4671)
  line L1512 (-41, 59.4671) -> (-36, 56.5803)
  line L1513 (-36, 56.5803) -> (-31, 59.4671)
  line L1514 (-24, 68.1273) -> (-29, 65.2406)
  line L1515 (-19, 65.2406) -> (-24, 68.1273)
  line L1516 (-19, 59.4671) -> (-19, 65.2406)
  line L1517 (-29, 65.2406) -> (-29, 59.4671)
  line L1518 (-29, 59.4671) -> (-24, 56.5803)
  line L1519 (-24, 56.5803) -> (-19, 59.4671)
  line L1520 (-12, 68.1273) -> (-17, 65.2406)
  line L1521 (-7, 65.2406) -> (-12, 68.1273)
  line L1522 (-7, 59.4671) -> (-7, 65.2406)
  line L1523 (-17, 65.2406) -> (-17, 59.4671)
  line L1524 (-17, 59.4671) -> (-12, 56.5803)
  line L1525 (-12, 56.5803) -> (-7, 59.4671)
  line L1526 (0, 68.1273) -> (-5, 65.2406)
  line L1527 (5, 65.2406) -> (0, 68.1273)
  line L1528 (5, 59.4671) -> (5, 65.2406)
  line L1529 (-5, 65.2406) -> (-5, 59.4671)
  line L1530 (-5, 59.4671) -> (0, 56.5803)
  line L1531 (0, 56.5803) -> (5, 59.4671)
  line L1532 (12, 68.1273) -> (7, 65.2406)
  line L1533 (17, 65.2406) -> (12, 68.1273)
  line L1534 (17, 59.4671) -> (17, 65.2406)
  line L1535 (7, 65.2406) -> (7, 59.4671)
  line L1536 (7, 59.4671) -> (12, 56.5803)
  line L1537 (12, 56.5803) -> (17, 59.4671)
  line L1538 (24, 68.1273) -> (19, 65.2406)
  line L1539 (29, 65.2406) -> (24, 68.1273)
  line L1540 (29, 59.4671) -> (29, 65.2406)
  line L1541 (19, 65.2406) -> (19, 59.4671)
  line L1542 (19, 59.4671) -> (24, 56.5803)
  line L1543 (24, 56.5803) -> (29, 59.4671)
  line L1544 (36, 68.1273) -> (31, 65.2406)
  line L1545 (41, 65.2406) -> (36, 68.1273)
  line L1546 (41, 59.4671) -> (41, 65.2406)
  line L1547 (31, 65.2406) -> (31, 59.4671)
  line L1548 (31, 59.4671) -> (36, 56.5803)
  line L1549 (36, 56.5803) -> (41, 59.4671)
  line L1550 (48, 68.1273) -> (43, 65.2406)
  line L1551 (53, 65.2406) -> (48, 68.1273)
  line L1552 (53, 59.4671) -> (53, 65.2406)
  line L1553 (43, 65.2406) -> (43, 59.4671)
  line L1554 (43, 59.4671) -> (48, 56.5803)
  line L1555 (48, 56.5803) -> (53, 59.4671)
  line L1556 (60, 68.1273) -> (55, 65.2406)
  line L1557 (65, 65.2406) -> (60, 68.1273)
  line L1558 (65, 59.4671) -> (65, 65.2406)
  line L1559 (55, 65.2406) -> (55, 59.4671)
  line L1560 (55, 59.4671) -> (60, 56.5803)
  line L1561 (60, 56.5803) -> (65, 59.4671)
  line L1562 (72, 68.1273) -> (67, 65.2406)
  line L1563 (77, 65.2406) -> (72, 68.1273)
  line L1564 (77, 59.4671) -> (77, 65.2406)
  line L1565 (67, 65.2406) -> (67, 59.4671)
  line L1566 (67, 59.4671) -> (72, 56.5803)
  line L1567 (72, 56.5803) -> (77, 59.4671)
  line L1568 (84, 68.1273) -> (79, 65.2406)
  line L1569 (89, 65.2406) -> (84, 68.1273)
  line L1570 (89, 59.4671) -> (89, 65.2406)
  line L1571 (79, 65.2406) -> (79, 59.4671)
  line L1572 (79, 59.4671) -> (84, 56.5803)
  line L1573 (84, 56.5803) -> (89, 59.4671)
  line L1574 (96, 68.1273) -> (91, 65.2406)
  line L1575 (101, 65.2406) -> (96, 68.1273)
  line L1576 (101, 59.4671) -> (101, 65.2406)
  line L1577 (91, 65.2406) -> (91, 59.4671)
  line L1578 (91, 59.4671) -> (96, 56.5803)
  line L1579 (96, 56.5803) -> (101, 59.4671)
  line L1580 (108, 68.1273) -> (103, 65.2406)
  line L1581 (113, 65.2406) -> (108, 68.1273)
  line L1582 (113, 59.4671) -> (113, 65.2406)
  line L1583 (103, 65.2406) -> (103, 59.4671)
  line L1584 (103, 59.4671) -> (108, 56.5803)
  line L1585 (108, 56.5803) -> (113, 59.4671)
  line L1586 (120, 68.1273) -> (115, 65.2406)
  line L1587 (125, 65.2406) -> (120, 68.1273)
  line L1588 (125, 59.4671) -> (125, 65.2406)
  line L1589 (115, 65.2406) -> (115, 59.4671)
  line L1590 (115, 59.4671) -> (120, 56.5803)
  line L1591 (120, 56.5803) -> (125, 59.4671)
  line L1592 (132, 68.1273) -> (127, 65.2406)
  line L1593 (137, 65.2406) -> (132, 68.1273)
  line L1594 (137, 59.4671) -> (137, 65.2406)
  line L1595 (127, 65.2406) -> (127, 59.4671)
  line L1596 (127, 59.4671) -> (132, 56.5803)
  line L1597 (132, 56.5803) -> (137, 59.4671)
  line L1598 (144, 68.1273) -> (139, 65.2406)
  line L1599 (149, 65.2406) -> (144, 68.1273)
  line L1600 (149, 59.4671) -> (149, 65.2406)
  line L1601 (139, 65.2406) -> (139, 59.4671)
  line L1602 (139, 59.4671) -> (144, 56.5803)
  line L1603 (144, 56.5803) -> (149, 59.4671)
  line L1604 (-66, 78.5196) -> (-71, 75.6329)
  line L1605 (-61, 75.6329) -> (-66, 78.5196)
  line L1606 (-61, 69.8594) -> (-61, 75.6329)
  line L1607 (-71, 75.6329) -> (-71, 69.8594)
  line L1608 (-71, 69.8594) -> (-66, 66.9726)
  line L1609 (-66, 66.9726) -> (-61, 69.8594)
  line L1610 (-54, 78.5196) -> (-59, 75.6329)
  line L1611 (-49, 75.6329) -> (-54, 78.5196)
  line L1612 (-49, 69.8594) -> (-49, 75.6329)
  line L1613 (-59, 75.6329) -> (-59, 69.8594)
  line L1614 (-59, 69.8594) -> (-54, 66.9726)
  line L1615 (-54, 66.9726) -> (-49, 69.8594)
  line L1616 (-42, 78.5196) -> (-47, 75.6329)
  line L1617 (-37, 75.6329) -> (-42, 78.5196)
  line L1618 (-37, 69.8594) -> (-37, 75.6329)
  line L1619 (-47, 75.6329) -> (-47, 69.8594)
  line L1620 (-47, 69.8594) -> (-42, 66.9726)
  line L1621 (-42, 66.9726) -> (-37, 69.8594)
  line L1622 (-30, 78.5196) -> (-35, 75.6329)
  line L1623 (-25, 75.6329) -> (-30, 78.5196)
  line L1624 (-25, 69.8594) -> (-25, 75.6329)
  line L1625 (-35, 75.6329) -> (-35, 69.8594)
  line L1626 (-35, 69.8594) -> (-30, 66.9726)
  line L1627 (-30, 66.9726) -> (-25, 69.8594)
  line L1628 (-18, 78.5196) -> (-23, 75.6329)
  line L1629 (-13, 75.6329) -> (-18, 78.5196)
  line L1630 (-13, 69.8594) -> (-13, 75.6329)
  line L1631 (-23, 75.6329) -> (-23, 69.8594)
  line L1632 (-23, 69.8594) -> (-18, 66.9726)
  line L1633 (-18, 66.9726) -> (-13, 69.8594)
  line L1634 (-6, 78.5196) -> (-11, 75.6329)
  line L1635 (-1, 75.6329) -> (-6, 78.5196)
  line L1636 (-1, 69.8594) -> (-1, 75.6329)
  line L1637 (-11, 75.6329) -> (-11, 69.8594)
  line L1638 (-11, 69.8594) -> (-6, 66.9726)
  line L1639 (-6, 66.9726) -> (-1, 69.8594)
  line L1640 (6, 78.5196) -> (1, 75.6329)
  line L1641 (11, 75.6329) -> (6, 78.5196)
  line L1642 (11, 69.8594) -> (11, 75.6329)
  line L1643 (1, 75.6329) -> (1, 69.8594)
  line L1644 (1, 69.8594) -> (6, 66.9726)
  line L1645 (6, 66.9726) -> (11, 69.8594)
  line L1646 (18, 78.5196) -> (13, 75.6329)
  line L1647 (23, 75.6329) -> (18, 78.5196)
  line L1648 (23, 69.8594) -> (23, 75.6329)
  line L1649 (13, 75.6329) -> (13, 69.8594)
  line L1650 (13, 69.8594) -> (18, 66.9726)
  line L1651 (18, 66.9726) -> (23, 69.8594)
  line L1652 (30, 78.5196) -> (25, 75.6329)
  line L1653 (35, 75.6329) -> (30, 78.5196)
  line L1654 (35, 69.8594) -> (35, 75.6329)
  line L1655 (25, 75.6329) -> (25, 69.8594)
  line L1656 (25, 69.8594) -> (30, 66.9726)
  line L1657 (30, 66.9726) -> (35, 69.8594)
  line L1658 (42, 78.5196) -> (37, 75.6329)
  line L1659 (47, 75.6329) -> (42, 78.5196)
  line L1660 (47, 69.8594) -> (47, 75.6329)
  line L1661 (37, 75.6329) -> (37, 69.8594)
  line L1662 (37, 69.8594) -> (42, 66.9726)
  line L1663 (42, 66.9726) -> (47, 69.8594)
  line L1664 (54, 78.5196) -> (49, 75.6329)
  line L1665 (59, 75.6329) -> (54, 78.5196)
  line L1666 (59, 69.8594) -> (59, 75.6329)
  line L1667 (49, 75.6329) -> (49, 69.8594)
  line L1668 (49, 69.8594) -> (54, 66.9726)
  line L1669 (54, 66.9726) -> (59, 69.8594)
  line L1670 (66, 78.5196) -> (61, 75.6329)
  line L1671 (71, 75.6329) -> (66, 78.5196)
  line L1672 (71, 69.8594) -> (71, 75.6329)
  line L1673 (61, 75.6329) -> (61, 69.8594)
  line L1674 (61, 69.8594) -> (66, 66.9726)
  line L1675 (66, 66.9726) -> (71, 69.8594)
  line L1676 (78, 78.5196) -> (73, 75.6329)
  line L1677 (83, 75.6329) -> (78, 78.5196)
  line L1678 (83, 69.8594) -> (83, 75.6329)
  line L1679 (73, 75.6329) -> (73, 69.8594)
  line L1680 (73, 69.8594) -> (78, 66.9726)
  line L1681 (78, 66.9726) -> (83, 69.8594)
  line L1682 (90, 78.5196) -> (85, 75.6329)
  line L1683 (95, 75.6329) -> (90, 78.5196)
  line L1684 (95, 69.8594) -> (95, 75.6329)
  line L1685 (85, 75.6329) -> (85, 69.8594)
  line L1686 (85, 69.8594) -> (90, 66.9726)
  line L1687 (90, 66.9726) -> (95, 69.8594)
  line L1688 (102, 78.5196) -> (97, 75.6329)
  line L1689 (107, 75.6329) -> (102, 78.5196)
  line L1690 (107, 69.8594) -> (107, 75.6329)
  line L1691 (97, 75.6329) -> (97, 69.8594)
  line L1692 (97, 69.8594) -> (102, 66.9726)
  line L1693 (102, 66.9726) -> (107, 69.8594)
  line L1694 (114, 78.5196) -> (109, 75.6329)
  line L1695 (119, 75.6329) -> (114, 78.5196)
  line L1696 (119, 69.8594) -> (119, 75.6329)
  line L1697 (109, 75.6329) -> (109, 69.8594)
  line L1698 (109, 69.8594) -> (114, 66.9726)
  line L1699 (114, 66.9726) -> (119, 69.8594)
  line L1700 (126, 78.5196) -> (121, 75.6329)
  line L1701 (131, 75.6329) -> (126, 78.5196)
  line L1702 (131, 69.8594) -> (131, 75.6329)
  line L1703 (121, 75.6329) -> (121, 69.8594)
  line L1704 (121, 69.8594) -> (126, 66.9726)
  line L1705 (126, 66.9726) -> (131, 69.8594)
  line L1706 (138, 78.5196) -> (133, 75.6329)
  line L1707 (143, 75.6329) -> (138, 78.5196)
  line L1708 (143, 69.8594) -> (143, 75.6329)
  line L1709 (133, 75.6329) -> (133, 69.8594)
  line L1710 (133, 69.8594) -> (138, 66.9726)
  line L1711 (138, 66.9726) -> (143, 69.8594)
  line L1712 (150, 78.5196) -> (145, 75.6329)
  line L1713 (155, 75.6329) -> (150, 78.5196)
  line L1714 (155, 69.8594) -> (155, 75.6329)
  line L1715 (145, 75.6329) -> (145, 69.8594)
  line L1716 (145, 69.8594) -> (150, 66.9726)
  line L1717 (150, 66.9726) -> (155, 69.8594)
  point P0 (-150, -72.7461)
  point P1 (-150, -72.7461)
  point P2 (-147.5, -68.416)
  point P3 (-145, -72.7461)
  point P4 (-150, -72.7461)
  point P5 (-150, -72.7461)
  point P6 (-138, -72.7461)
  point P7 (-138, -72.7461)
  point P8 (-135.5, -68.416)
  point P9 (-133, -72.7461)
  point P10 (-138, -72.7461)
  point P11 (-138, -72.7461)
  point P12 (-126, -72.7461)
  point P13 (-126, -72.7461)
  point P14 (-123.5, -68.416)
  point P15 (-121, -72.7461)
  point P16 (-126, -72.7461)
  point P17 (-126, -72.7461)
  point P18 (-114, -72.7461)
  point P19 (-114, -72.7461)
  point P20 (-111.5, -68.416)
  point P21 (-109, -72.7461)
  point P22 (-114, -72.7461)
  point P23 (-114, -72.7461)
  point P24 (-102, -72.7461)
  point P25 (-102, -72.7461)
  point P26 (-99.5, -68.416)
  point P27 (-97, -72.7461)
  point P28 (-102, -72.7461)
  point P29 (-102, -72.7461)
  point P30 (-90, -72.7461)
  point P31 (-90, -72.7461)
  point P32 (-87.5, -68.416)
  point P33 (-85, -72.7461)
  point P34 (-90, -72.7461)
  point P35 (-90, -72.7461)
  point P36 (-78, -72.7461)
  point P37 (-78, -72.7461)
  point P38 (-75.5, -68.416)
  point P39 (-73, -72.7461)
  point P40 (-78, -72.7461)
  point P41 (-78, -72.7461)
  point P42 (-66, -72.7461)
  point P43 (-66, -72.7461)
  point P44 (-63.5, -68.416)
  point P45 (-61, -72.7461)
  point P46 (-66, -72.7461)
  point P47 (-66, -72.7461)
  point P48 (-54, -72.7461)
  point P49 (-54, -72.7461)
  point P50 (-51.5, -68.416)
  point P51 (-49, -72.7461)
  point P52 (-54, -72.7461)
  point P53 (-54, -72.7461)
  point P54 (-42, -72.7461)
  point P55 (-42, -72.7461)
  point P56 (-39.5, -68.416)
  point P57 (-37, -72.7461)
  point P58 (-42, -72.7461)
  point P59 (-42, -72.7461)
  point P60 (-30, -72.7461)
  point P61 (-30, -72.7461)
  point P62 (-27.5, -68.416)
  point P63 (-25, -72.7461)
  point P64 (-30, -72.7461)
  point P65 (-30, -72.7461)
  point P66 (-18, -72.7461)
  point P67 (-18, -72.7461)
  point P68 (-15.5, -68.416)
  point P69 (-13, -72.7461)
  point P70 (-18, -72.7461)
  point P71 (-18, -72.7461)
  point P72 (-6, -72.7461)
  point P73 (-6, -72.7461)
  point P74 (-3.5, -68.416)
  point P75 (-1, -72.7461)
  point P76 (-6, -72.7461)
  point P77 (-6, -72.7461)
  point P78 (6, -72.7461)
  point P79 (6, -72.7461)
  point P80 (8.5, -68.416)
  point P81 (11, -72.7461)
  point P82 (6, -72.7461)
  point P83 (6, -72.7461)
  point P84 (18, -72.7461)
  point P85 (18, -72.7461)
  point P86 (20.5, -68.416)
  point P87 (23, -72.7461)
  point P88 (18, -72.7461)
  point P89 (18, -72.7461)
  point P90 (30, -72.7461)
  point P91 (30, -72.7461)
  point P92 (32.5, -68.416)
  point P93 (35, -72.7461)
  point P94 (30, -72.7461)
  point P95 (30, -72.7461)
  point P96 (42, -72.7461)
  point P97 (42, -72.7461)
  point P98 (44.5, -68.416)
  point P99 (47, -72.7461)
  point P100 (42, -72.7461)
  point P101 (42, -72.7461)
  point P102 (54, -72.7461)
  point P103 (54, -72.7461)
  point P104 (56.5, -68.416)
  point P105 (59, -72.7461)
  point P106 (54, -72.7461)
  point P107 (54, -72.7461)
  point P108 (66, -72.7461)
  point P109 (66, -72.7461)
  point P110 (68.5, -68.416)
  point P111 (71, -72.7461)
  point P112 (66, -72.7461)
  point P113 (66, -72.7461)
  point P114 (-144, -62.3538)
  point P115 (-144, -62.3538)
  point P116 (-141.5, -58.0237)
  point P117 (-139, -62.3538)
  point P118 (-144, -62.3538)
  point P119 (-144, -62.3538)
  point P120 (-132, -62.3538)
  point P121 (-132, -62.3538)
  point P122 (-129.5, -58.0237)
  point P123 (-127, -62.3538)
  point P124 (-132, -62.3538)
  point P125 (-132, -62.3538)
  point P126 (-120, -62.3538)
  point P127 (-120, -62.3538)
  point P128 (-117.5, -58.0237)
  point P129 (-115, -62.3538)
  point P130 (-120, -62.3538)
  point P131 (-120, -62.3538)
  point P132 (-108, -62.3538)
  point P133 (-108, -62.3538)
  point P134 (-105.5, -58.0237)
  point P135 (-103, -62.3538)
  point P136 (-108, -62.3538)
  point P137 (-108, -62.3538)
  point P138 (-96, -62.3538)
  point P139 (-96, -62.3538)
  point P140 (-93.5, -58.0237)
  point P141 (-91, -62.3538)
  point P142 (-96, -62.3538)
  point P143 (-96, -62.3538)
  point P144 (-84, -62.3538)
  point P145 (-84, -62.3538)
  point P146 (-81.5, -58.0237)
  point P147 (-79, -62.3538)
  point P148 (-84, -62.3538)
  point P149 (-84, -62.3538)
  point P150 (-72, -62.3538)
  point P151 (-72, -62.3538)
  point P152 (-69.5, -58.0237)
  point P153 (-67, -62.3538)
  point P154 (-72, -62.3538)
  point P155 (-72, -62.3538)
  point P156 (-60, -62.3538)
  point P157 (-60, -62.3538)
  point P158 (-57.5, -58.0237)
  point P159 (-55, -62.3538)
  point P160 (-60, -62.3538)
  point P161 (-60, -62.3538)
  point P162 (-48, -62.3538)
  point P163 (-48, -62.3538)
  point P164 (-45.5, -58.0237)
  point P165 (-43, -62.3538)
  point P166 (-48, -62.3538)
  point P167 (-48, -62.3538)
  point P168 (-36, -62.3538)
  point P169 (-36, -62.3538)
  point P170 (-33.5, -58.0237)
  point P171 (-31, -62.3538)
  point P172 (-36, -62.3538)
  point P173 (-36, -62.3538)
  point P174 (-24, -62.3538)
  point P175 (-24, -62.3538)
  point P176 (-21.5, -58.0237)
  point P177 (-19, -62.3538)
  point P178 (-24, -62.3538)
  point P179 (-24, -62.3538)
  point P180 (-12, -62.3538)
  point P181 (-12, -62.3538)
  point P182 (-9.5, -58.0237)
  point P183 (-7, -62.3538)
  point P184 (-12, -62.3538)
  point P185 (-12, -62.3538)
  point P186 (0, -62.3538)
  point P187 (0, -62.3538)
  point P188 (2.5, -58.0237)
  point P189 (5, -62.3538)
  point P190 (0, -62.3538)
  point P191 (0, -62.3538)
  point P192 (12, -62.3538)
  point P193 (12, -62.3538)
  point P194 (14.5, -58.0237)
  point P195 (17, -62.3538)